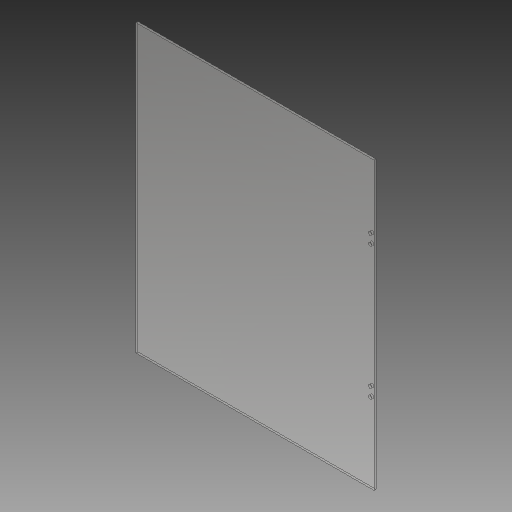
# Autodesk Inventor part: Porte
Saved by Autodesk Inventor 2017 (Build 210142000, 142)
## iProperties
Company: FABLAB Frenchmakers
Part Number: Porte
Project: 1400-PopCorn Machine
Material: Plastique PMMA
Catalog Web Link: http://www.frenchmakers.com/
Document SubType Name: Modeling
Designer: FABLAB Frenchmakers
Density: 1.188 g/cm^3
Appearance: Polycarbonate - Transparent
Stock Number: 1400-04-06
Author: Adrien MARY
Autodesk Inventor part; units mm, degrees
ref_plane "YZ Plane" through (0, 0, 0) normal (1, 0, 0) x (0, 1, 0)
ref_plane "XZ Plane" through (0, 0, 0) normal (0, 1, 0) x (-1, 0, 0)
ref_plane "XY Plane" through (0, 0, 0) normal (0, 0, 1) x (1, 0, 0)
sketch "Esquisse1" plane through (0, 0, 0) normal (0, 0, 1) x (1, 0, 0)
  line L0 (-179.9, -216) -> (179.9, -216)
  line L1 (179.9, -216) -> (179.9, 216)
  line L2 (179.9, 216) -> (-179.9, 216)
  line L3 (-179.9, 216) -> (-179.9, -216)
  line L4 (-179.9, -216) -> (179.9, 216) construction
  line L5 (179.9, -216) -> (-179.9, 216) construction
  point P0 (0, 0)
  dimension "Largueur_porte" = 359.8
  dimension "Hauteur_porte" = 432
  constraints: 12 end point, 2 midpoint, 2 parallel, 1 horizontal, 1 perpendicular
  measures "Largueur_porte" distance of L1.end L2.end
  measures "Hauteur_porte" distance of L2.end L0.start
extrude "Embase" add sketch "Esquisse1" along normal mid plane 3
sketch "Esquisse2" plane through (0, 0, -1.5) normal (0, 0, -1) x (-1, 0, 0)
  ellipse E0 centre (-178.8362, -97) end of major axis (-178.8362, -94.5) minor radius 1.7678 projected
  ellipse E1 centre (-178.8362, -83) end of major axis (-178.8362, -80.5) minor radius 1.7678 projected
  ellipse E2 centre (-178.8362, 117) end of major axis (-178.8362, 119.5) minor radius 1.7678 projected
  ellipse E3 centre (-178.8362, 103) end of major axis (-178.8362, 105.5) minor radius 1.7678 projected
  point P0 (0, 0)
  point P1 (-173.9322, 117)
  point P2 (-173.9322, 103)
  point P3 (-173.9322, -83)
  point P4 (-173.9322, -97)
  constraints: 4 other
hole "Perçage1" at (173.9322, 117, -1.5) at (173.9322, 103, -1.5) at (173.9322, -83, -1.5) at (173.9322, -97, -1.5) direction (0, 0, 1) diameter 5.5 end through all clearance for "Vis à tête plate fraisée ISO 2009/7046" size "M5" standard "ISO"
